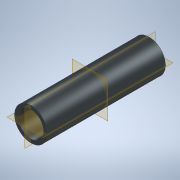
# Autodesk Inventor part: switchHangingPipe
Saved by Autodesk Inventor 2020.2 (Build 242310000, 310)
## iProperties
Created: 2020-01-06
Part Number: switchHangingPipe
Material: Iron, Gray
Document SubType Name: Modeling
Designer: steele
Density: 7.15 g/cm^3
Appearance: Iron Gray
Author: steele
Autodesk Inventor part; units mm, degrees
sketch "Sketch1" plane through (0, 0, 0) normal (0, 0, 1) x (1, 0, 0)
  circle A0 centre (0, 0) radius 16.51
  circle A1 centre (0, 0) radius 21.082
  dimension "d0" = 33.02
  dimension "d1" = 42.164
  constraints: 2 centre point, 2 coincident
  measures "d0" diameter of A0
  measures "d1" diameter of A1
extrude "Extrusion1" add sketch "Sketch1" along normal mid plane 152.4
body "Solid1"
